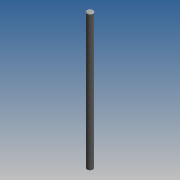
# Autodesk Inventor part: P113
Saved by Autodesk Inventor 2019 (Build 230136000, 136)
## iProperties
Created: 2016-11-02
Part Number: P113
Material: Generic
Document SubType Name: Modeling
Designer: serge.amoos
Density: 1 g/cm^3
Appearance: Par défaut
Description: Tige filetée M3
Author: serge.amoos
Autodesk Inventor part; units mm, degrees
ref_plane "YZ Plane" through (0, 0, 0) normal (1, 0, 0) x (0, 1, 0)
ref_plane "XZ Plane" through (0, 0, 0) normal (0, 1, 0) x (-1, 0, 0)
ref_plane "XY Plane" through (0, 0, 0) normal (0, 0, 1) x (1, 0, 0)
sketch "Sketch1" plane through (0, 0, 0) normal (0, 0, 1) x (1, 0, 0)
  circle A0 centre (0, 0) radius 1.5
  dimension "d0" = 3
  constraints: 1 centre point, 1 coincident
  measures "d0" diameter of A0
extrude "Extrusion1" add sketch "Sketch1" along normal blind 70
chamfer "Chamfer1" distance 0.3 angle 45 2 edges at (-1.5, 0, 70) (-1.5, 0, 0)
thread "Thread1" size "M3x0.5" class "6g" standard "ISO Metric profile" full length
body "Solid1"
